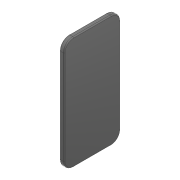
# Autodesk Inventor part: Phone
Saved by Autodesk Inventor 2020.2 (Build 242310000, 310)
## iProperties
Created: 2020-01-10
Part Number: Phone
Material: Glass
Document SubType Name: Modeling
Designer: webbg
Density: 2.18 g/cm^3
Appearance: Smooth - Black
Company: FTC VISION 14189
Author: webbg
Autodesk Inventor part; units mm, degrees
ref_plane "YZ Plane" through (0, 0, 0) normal (1, 0, 0) x (0, 1, 0)
ref_plane "XZ Plane" through (0, 0, 0) normal (0, 1, 0) x (-1, 0, 0)
ref_plane "XY Plane" through (0, 0, 0) normal (0, 0, 1) x (1, 0, 0)
sketch "Actobotics Pattern" plane through (0, 0, 0) normal (0, 0, 1) x (1, 0, 0)
  circle A0 centre (12.1352, -23.7422) radius 1.778
  circle A1 centre (9.525, -16.8274) radius 2.032
  circle A2 centre (19.05, -16.8274) radius 6.35
  circle A3 centre (19.05, -7.0484) radius 1.778
  circle A4 centre (19.05, -26.6064) radius 1.778
  circle A5 centre (25.9648, -9.9126) radius 1.778
  circle A6 centre (31.1852, -23.7422) radius 1.778
  circle A7 centre (24.6072, -30.2753) radius 1.778
  circle A8 centre (32.5428, -30.2753) radius 1.778
  circle A9 centre (28.575, -16.8274) radius 2.032
  circle A10 centre (25.9648, -23.7422) radius 1.778
  circle A11 centre (12.1352, -9.9126) radius 1.778
  circle A12 centre (31.1852, -9.9126) radius 1.778
  circle A13 centre (24.6296, -3.3571) radius 1.778
  circle A14 centre (32.5204, -3.3571) radius 1.778
  circle A15 centre (6.9148, -23.7422) radius 1.778
  circle A16 centre (6.9148, -9.9126) radius 1.778
  circle A17 centre (13.4928, -30.2753) radius 1.778
  circle A18 centre (13.4704, -3.3571) radius 1.778
  circle A19 centre (5.5796, -3.3571) radius 1.778
  circle A20 centre (5.5572, -30.2753) radius 1.778
  point P0 (12.1352, -9.9126)
  point P1 (9.271, -16.8274)
  point P2 (25.9648, -23.7422)
  point P3 (28.829, -16.8274)
  dimension "d2" = 12.7
  dimension "d7" = 360
  dimension "d8" = 3.556
  dimension "d9" = 3.556
  dimension "d10" = 3.556
  dimension "d11" = 3.556
  dimension "d12" = 3.556
  dimension "d13" = 3.556
  dimension "d15" = 3.556
  dimension "d16" = 3.556
  dimension "d17" = 3.556
  dimension "d22" = 4.064
  dimension "d23" = 4.064
  dimension "d24" = 3.556
  dimension "d25" = 3.556
  dimension "d26" = 3.556
  dimension "d27" = 3.556
  dimension "d28" = 3.556
  dimension "d29" = 3.556
  dimension "d30" = 3.556
  dimension "d31" = 3.556
  measures "d2" diameter of A2
  measures "d8" diameter of A3
  measures "d9" diameter of A5
  measures "d10" diameter of A10
  measures "d11" diameter of A4
  measures "d12" diameter of A0
  measures "d13" diameter of A11
  measures "d15" diameter of A19
  measures "d16" diameter of A8
  measures "d17" diameter of A20
  measures "d22" diameter of A1
  measures "d23" diameter of A9
  measures "d24" diameter of A15
  measures "d25" diameter of A6
  measures "d26" diameter of A12
  measures "d27" diameter of A16
  measures "d28" diameter of A17
  measures "d29" diameter of A7
  measures "d30" diameter of A13
  measures "d31" diameter of A18
sketch "REV Hub Screw Pattern" plane through (0, 0, 0) normal (0, 0, 1) x (1, 0, 0)
  circle A0 centre (7.5, 7.5) radius 1.7
  circle A1 centre (7.5, 135.5) radius 1.7
  circle A2 centre (95.5, 135.5) radius 1.7
  circle A3 centre (95.5, 7.5) radius 1.7
  line L0 (2.9959, 0) -> (100.0041, 0)
  ellipse E0 centre (3.0041, 3.0041) end of major axis (0.877, 0.877) minor radius 3 (0, 2.9959) -> (2.9959, 0) ccw
  line L1 (0, 2.9959) -> (0, 140.0041)
  ellipse E1 centre (3.0041, 139.9959) end of major axis (0.877, 142.123) minor radius 3 (2.9959, 143) -> (0, 140.0041) ccw
  line L2 (100.0041, 143) -> (2.9959, 143)
  ellipse E2 centre (99.9959, 139.9959) end of major axis (97.8687, 137.8687) minor radius 3 (103, 140.0041) -> (100.0041, 143) ccw
  line L3 (103, 2.9959) -> (103, 140.0041)
  ellipse E3 centre (99.9959, 3.0041) end of major axis (102.123, 0.877) minor radius 3 (100.0041, 0) -> (103, 2.9959) ccw
  point P0 (0, 0)
  point P1 (0, 0)
sketch "Sketch2" plane through (0, 0, 0) normal (1, 0, 0) x (0, 1, 0)
  line L0 (12.7, 0) -> (139.7, 0)
  line L1 (152.4, -12.7) -> (152.4, -63.5)
  line L2 (139.7, -76.2) -> (12.7, -76.2)
  line L3 (0, -63.5) -> (0, -12.7)
  arc A0 (152.4, -12.7) -> (139.7, 0) centre (139.7, -12.7) ccw
  arc A1 (12.7, 0) -> (0, -12.7) centre (12.7, -12.7) ccw
  arc A2 (0, -63.5) -> (12.7, -76.2) centre (12.7, -63.5) ccw
  arc A3 (139.7, -76.2) -> (152.4, -63.5) centre (139.7, -63.5) ccw
  point P0 (0, 0)
  point P1 (152.4, -76.2)
  point P2 (152.4, 0)
  point P3 (0, -76.2)
  dimension "d34" = 152.4
  dimension "d35" = 76.2
  dimension "d36" = 12.7
  constraints: 8 end point, 8 point on circle, 8 point on line, 8 tangent, 4 centre point, 3 equal radius, 2 parallel, 1 horizontal, 1 perpendicular
  measures "d34" distance of point (152.4, -76.2) point (0, -76.2)
  measures "d35" distance of point (152.4, 0) point (152.4, -76.2)
  measures "d36" radius of A0
extrude "Extrusion1" add sketch "Sketch2" along normal blind 6.35
fillet "Fillet1" radius 1.27 16 edges at (6.35, 3.7197, -3.7197) (6.35, 0, -38.1) (6.35, 3.7197, -72.4803) (6.35, 76.2, -76.2) (6.35, 148.6803, -72.4803) (6.35, 152.4, -38.1) (6.35, 148.6803, -3.7197) (6.35, 76.2, 0) (0, 3.7197, -3.7197) (0, 0, -38.1) (0, 3.7197, -72.4803) (0, 76.2, -76.2) (0, 148.6803, -72.4803) (0, 152.4, -38.1) (0, 148.6803, -3.7197) (0, 76.2, 0)
body "Solid1"
